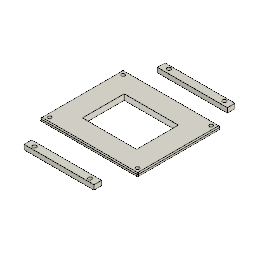
LCD Bezel 2.4in clamp-down v2 (Autodesk Fusion 360 design; units mm, degrees)
Autodesk Fusion 360 part; units mm, degrees
note: some values were not read from the file. Set by a fixed rule: which sketch regions a step uses.
sketch "Sketch1" plane through (0, 0, 0) normal (0, 0, 1) x (1, 0, 0)
  line L0 (-50.5, 43) -> (50.5, 43)
  line L1 (50.5, 43) -> (50.5, -43)
  line L2 (50.5, -43) -> (-50.5, -43)
  line L3 (-50.5, -43) -> (-50.5, 43)
  line L4 (-50.5, 43) -> (50.5, -43) construction
  line L5 (50.5, 43) -> (-50.5, -43) construction
  line L6 (25, 18.6) -> (-25, 18.6)
  line L7 (-25, 18.6) -> (-25, -18.6)
  line L8 (-25, -18.6) -> (25, -18.6)
  line L9 (25, -18.6) -> (25, 18.6)
  line L10 (25, 18.6) -> (-25, -18.6) construction
  line L11 (-25, 18.6) -> (25, -18.6) construction
  circle A0 centre (-45.5, 38) radius 5 construction
  circle A1 centre (-45.5, 38) radius 1.815
  line L12 (0, 55) -> (0, -45) construction
  line L13 (-60, 0) -> (80, 0) construction
  circle A2 centre (45.5, 38) radius 1.815
  circle A3 centre (45.5, -38) radius 1.815
  circle A4 centre (-45.5, -38) radius 1.815
  dimension "d1" = 101
  dimension "d2" = 86
  dimension "d3" = 50
  dimension "d4" = 37.2
  dimension "d5" = 5
  dimension "d6" = 3.63
  constraint perpendicular L0 L1
  constraint parallel L0 L2
  constraint parallel L1 L3
  constraint horizontal L0
  constraint coincident L4 origin
  constraint coincident L5 origin
  constraint perpendicular L6 L7
  constraint parallel L6 L8
  constraint parallel L7 L9
  constraint horizontal L6
  constraint coincident L10 origin
  constraint coincident L11 origin
  constraint tangent L3 A0
  constraint tangent L0 A0
  constraint concentric A0 A1
  constraint perpendicular L2 L12
  constraint perpendicular L3 L13
  constraint symmetric A1 L12 A2
  constraint symmetric A1 L13 A4
  constraint symmetric L13 A2 A3
  measures "d1" distance of L1.end L2.end
  measures "d2" distance of L0.end L1.end
  measures "d3" distance of L7.end L8.end
  measures "d4" distance of L6.end L7.end
  measures "d5" radius of A0
  measures "d6" diameter of A1
  measures "d14" distance of L0.start
extrude "Extrude1" add sketch "Sketch1" along normal blind 3 makes body 1
chamfer "Chamfer1" distance 3 angle 45 4 edges at (-25, 0, 3) (0, 18.6, 3) (25, 0, 3) (0, -18.6, 3) on bodies 1
sketch "Sketch2" plane through (-50.5, 0, 0) normal (-1, 0, 0) x (0, -1, 0)
  line L0 (-43, 0) -> (43, 0)
  line L1 (43, 0) -> (43, 3)
  line L2 (43, 3) -> (-43, 3)
  line L3 (-43, 3) -> (-43, 0)
fillet "Fillet1" radius 1 3 edges at (0, -43, 3) (0, 43, 3) (50.5, 0, 3) on bodies 1
sketch "Sketch3" plane through (0, 0, 0) normal (0, 0, 1) x (1, 0, 0)
  line L0 (-25.3857, -13.813) -> (-25.3857, 46.187) construction
  line L1 (25, 18.6) -> (25, -18.6)
  line L2 (25, -13.1739) -> (25, 45.4) construction
  line L3 (-34.2857, 33.1645) -> (-34.2857, -36.2651) construction
  line L4 (38.2, 40.4) -> (38.2, -34.6) construction
  line L5 (-25.3857, 18.7093) -> (64.6852, 18.7093) construction
  line L6 (60, 27.4093) -> (56.9479, 27.4093) construction
  line L7 (56.9479, 27.4093) -> (-67.0893, 27.4093) construction
  line L8 (60, -25.5) -> (-63.5008, -25.5) construction
  line L9 (25, -18.6) -> (-75, -18.6) construction
  line L10 (-34.2857, 0) -> (-38.2857, 0)
  line L11 (-38.2857, 0) -> (-38.2857, -5)
  line L12 (-38.2857, -5) -> (-34.2857, -5)
  line L13 (-34.2857, -5) -> (-34.2857, 0)
  line L14 (-34.2857, 0) -> (-38.2857, 0)
  line L15 (-38.2857, 0) -> (-38.2857, 5)
  line L16 (-38.2857, 5) -> (-34.2857, 5)
  line L17 (-34.2857, 5) -> (-34.2857, 0)
  line L18 (38.2, -25.5) -> (42.2, -25.5)
  line L19 (42.2, -25.5) -> (42.2, -10.5)
  line L20 (42.2, -10.5) -> (38.2, -10.5)
  line L21 (38.2, -10.5) -> (38.2, -25.5)
  line L22 (38.2, 27.4093) -> (42.2, 27.4093)
  line L23 (42.2, 27.4093) -> (42.2, 12.4093)
  line L24 (42.2, 12.4093) -> (38.2, 12.4093)
  line L25 (38.2, 12.4093) -> (38.2, 27.4093)
  line L26 (-34.2857, 27.4093) -> (-19.2857, 27.4093)
  line L27 (-19.2857, 27.4093) -> (-19.2857, 34.4093)
  line L28 (-19.2857, 34.4093) -> (-34.2857, 34.4093)
  line L29 (-34.2857, 34.4093) -> (-34.2857, 27.4093)
  line L30 (38.2, 27.4093) -> (23.2, 27.4093)
  line L31 (23.2, 27.4093) -> (23.2, 34.4093)
  line L32 (23.2, 34.4093) -> (38.2, 34.4093)
  line L33 (38.2, 34.4093) -> (38.2, 27.4093)
  line L34 (-34.2857, -25.5) -> (-19.2857, -25.5)
  line L35 (-19.2857, -25.5) -> (-19.2857, -32.5)
  line L36 (-19.2857, -32.5) -> (-34.2857, -32.5)
  line L37 (-34.2857, -32.5) -> (-34.2857, -25.5)
  line L38 (38.2, -25.5) -> (23.2, -25.5)
  line L39 (23.2, -25.5) -> (23.2, -32.5)
  line L40 (23.2, -32.5) -> (38.2, -32.5)
  line L41 (38.2, -32.5) -> (38.2, -25.5)
  line L42 (38.2, -25.5) -> (42.2, -25.5)
  line L43 (42.2, -25.5) -> (42.2, -30.5)
  line L44 (40.2, -32.5) -> (38.2, -32.5)
  line L45 (38.2, -32.5) -> (38.2, -25.5)
  line L46 (38.2, 27.4093) -> (42.2, 27.4093)
  line L47 (42.2, 27.4093) -> (42.2, 32.4093)
  line L48 (40.2, 34.4093) -> (38.2, 34.4093)
  line L49 (38.2, 34.4093) -> (38.2, 27.4093)
  line L50 (55, 0) -> (-65, 0) construction
  arc A0 (42.2, 32.4093) -> (40.2, 34.4093) centre (40.2, 32.4093) ccw
  arc A1 (40.2, -32.5) -> (42.2, -30.5) centre (40.2, -30.5) ccw
  dimension "d11" = 8.9
  dimension "d12" = 13.2
  dimension "d13" = 8.7
  dimension "d14" = 6.9
  dimension "d18" = 4
  dimension "d19" = 4
  dimension "d20" = 15
  dimension "d21" = 15
  dimension "d22" = 4
  dimension "d24" = 15
  dimension "d25" = 7
  dimension "d26" = 15
  dimension "d27" = 15
  dimension "d28" = 7
  dimension "d29" = 15
  dimension "d30" = 7
  dimension "d31" = 7
  dimension "d32" = 4
  dimension "d33" = 4
  dimension "d34" = 7
  dimension "d61" = 7
  dimension "d67" = 124.0372
  dimension "d75" = 2
  dimension "d76" = 2
  dimension "d79" = 4
  constraint vertical L0
  constraint coincident L1 L2.start
  constraint parallel L1 L2
  constraint vertical L3
  constraint vertical L4
  constraint coincident L0 L5.start
  constraint perpendicular L0 L5
  constraint horizontal L6
  constraint parallel L6 L7
  constraint horizontal L8
  constraint coincident L1.end L9.start
  constraint perpendicular L1 L9
  constraint horizontal L10
  constraint vertical L11
  constraint horizontal L12
  constraint vertical L13
  constraint coincident L3 L10.start
  constraint horizontal L14
  constraint vertical L15
  constraint horizontal L16
  constraint vertical L17
  constraint horizontal L18
  constraint vertical L19
  constraint horizontal L20
  constraint vertical L21
  constraint coincident L4 L18.start
  constraint coincident L8 L18.start
  constraint horizontal L22
  constraint vertical L23
  constraint horizontal L24
  constraint vertical L25
  constraint coincident L4 L22.start
  constraint coincident L7 L22.start
  constraint horizontal L26
  constraint vertical L27
  constraint horizontal L28
  constraint vertical L29
  constraint coincident L3 L26.start
  constraint coincident L7 L26.start
  constraint horizontal L30
  constraint vertical L31
  constraint horizontal L32
  constraint vertical L33
  constraint horizontal L34
  constraint vertical L35
  constraint horizontal L36
  constraint vertical L37
  constraint coincident L3 L34.start
  constraint coincident L8 L34.start
  constraint horizontal L38
  constraint vertical L39
  constraint horizontal L40
  constraint vertical L41
  constraint horizontal L42
  constraint vertical L43
  constraint horizontal L44
  constraint vertical L45
  constraint horizontal L46
  constraint vertical L47
  constraint horizontal L48
  constraint vertical L49
  constraint horizontal L50
  constraint tangent L47 A0
  constraint tangent L48 A0
  constraint tangent L44 A1
  constraint tangent L43 A1
  measures "d11" distance of L0 L3
  measures "d12" distance of L2 L4
  measures "d13" distance of L5 L7
  measures "d14" distance of L8 L9
  measures "d18" distance of L10.start L10.end
  measures "d19" distance of L18.start L18.end
  measures "d20" distance of L18.start L20.end
  measures "d21" distance of L22.start L24.end
  measures "d22" distance of L22.start L22.end
  measures "d24" distance of L26.start L26.end
  measures "d25" distance of L22.start L32.end
  measures "d26" distance of L22.start L30.end
  measures "d27" distance of L34.start L34.end
  measures "d28" distance of L34.start L36.end
  measures "d29" distance of L18.start L38.end
  measures "d30" distance of L18.start L40.end
  measures "d31" distance of L18.start L40.end
  measures "d32" distance of L18.start L18.end
  measures "d33" distance of L22.start L22.end
  measures "d34" distance of L22.start L32.end
  measures "d61" distance of L26 L28
  measures "d67" distance of L6.end L7.end
  measures "d75" radius of A0
  measures "d76" radius of A1
  measures "d79" distance of L3 L11
extrude "Extrude2" add sketch "Sketch3" against normal blind 6.2 bodies 1
fillet "Fillet2" radius 1 2 edges at (50.5, 43, 1) (50.2071, 42.7071, 2.7071) on bodies 1
fillet "Fillet3" radius 1 2 edges at (50.5, -43, 1) (50.2071, -42.7071, 2.7071) on bodies 1
sketch "Sketch4" plane through (0, -25.5, 0) normal (0, 1, 0) x (-1, 0, 0)
  line L0 (-23.2, 0) -> (-38.2, 0)
  line L1 (-38.2, 0) -> (-38.2, -6.2)
  line L2 (-38.2, -6.2) -> (-23.2, -6.2)
  line L3 (-23.2, -6.2) -> (-23.2, 0)
  line L4 (-23.2, -6.2) -> (-38.2, -6.2)
  line L5 (-38.2, -6.2) -> (-38.2, -3.2)
  line L6 (-38.2, -3.2) -> (-23.2, -3.2)
  line L7 (-23.2, -3.2) -> (-23.2, -6.2)
  dimension "d40" = 3
  constraint horizontal L4
  constraint vertical L5
  constraint horizontal L6
  constraint vertical L7
  constraint coincident L2.end L3.start
  measures "d40" distance of L2.end L6.end
fillet "Fillet4" radius 1 5 edges at (-50.5, 43, 1) (-50.5, 42.7071, 2.7071) (-50.5, 0, 3) (-50.5, -42.7071, 2.7071) (-50.5, -43, 1) on bodies 1
sketch "Sketch5" plane through (0, -25.5, 0) normal (0, 1, 0) x (-1, 0, 0)
  line L0 (34.2857, 0) -> (19.2857, 0)
  line L1 (19.2857, 0) -> (19.2857, -6.2)
  line L2 (19.2857, -6.2) -> (34.2857, -6.2)
  line L3 (34.2857, -6.2) -> (34.2857, 0)
  line L4 (34.2857, -6.2) -> (19.2857, -6.2)
  line L5 (19.2857, -6.2) -> (19.2857, -3.2)
  line L6 (19.2857, -3.2) -> (34.2857, -3.2)
  line L7 (34.2857, -3.2) -> (34.2857, -6.2)
  circle A0 centre (27.0136, -7.0821) radius 1090.7798
  dimension "d43" = 3
  constraint horizontal L4
  constraint vertical L5
  constraint horizontal L6
  constraint vertical L7
  constraint coincident L2.end L3.start
  measures "d43" distance of L2.end L6.end
sketch "Sketch6" plane through (0, 27.4093, 0) normal (0, -1, 0) x (1, 0, 0)
  line L0 (-19.2857, 0) -> (-34.2857, 0)
  line L1 (-34.2857, 0) -> (-34.2857, -6.2)
  line L2 (-34.2857, -6.2) -> (-19.2857, -6.2)
  line L3 (-19.2857, -6.2) -> (-19.2857, 0)
  line L4 (-19.2857, -6.2) -> (-34.2857, -6.2)
  line L5 (-34.2857, -6.2) -> (-34.2857, -3.2)
  line L6 (-34.2857, -3.2) -> (-19.2857, -3.2)
  line L7 (-19.2857, -3.2) -> (-19.2857, -6.2)
  dimension "d46" = 3
  constraint horizontal L4
  constraint vertical L5
  constraint horizontal L6
  constraint vertical L7
  constraint coincident L1 L5.end
  constraint coincident L2.end L3.start
  measures "d46" distance of L2.end L6.end
sketch "Sketch8" plane through (0, 0, -6.2) normal (0, 0, -1) x (1, 0, 0)
  line L0 (38.2, 25.5) -> (37.2, 25.5)
  line L1 (37.2, 25.5) -> (37.2, 29.5)
  line L2 (37.2, 29.5) -> (38.2, 29.5)
  line L3 (38.2, 29.5) -> (38.2, 25.5)
  line L4 (42.2, 10.5) -> (42.2, 30.5)
  arc A0 (42.2, 30.5) -> (40.2, 32.5) centre (40.2, 30.5) ccw
  line L5 (40.2, 32.5) -> (23.2, 32.5)
  line L6 (23.2, 32.5) -> (23.2, 25.5)
  line L7 (23.2, 25.5) -> (38.2, 25.5)
  line L8 (38.2, 25.5) -> (38.2, 10.5)
  line L9 (38.2, 10.5) -> (42.2, 10.5)
  dimension "d52" = 1
  constraint horizontal L0
  constraint vertical L1
  constraint horizontal L2
  constraint vertical L3
  measures "d52" distance of L0.start L0.end
sketch "Sketch10" plane through (0, 27.4093, 0) normal (0, -1, 0) x (1, 0, 0)
  line L0 (38.2, 0) -> (23.2, 0)
  line L1 (23.2, 0) -> (23.2, -6.2)
  line L2 (23.2, -6.2) -> (38.2, -6.2)
  line L3 (23.2, -6.2) -> (37.2, -6.2)
  line L4 (37.2, -6.2) -> (37.2, -3.2)
  line L5 (37.2, -3.2) -> (23.2, -3.2)
  line L6 (23.2, -3.2) -> (23.2, -6.2)
  line L7 (38.2, -6.2) -> (38.2, 0)
  dimension "d58" = 3
  constraint horizontal L3
  constraint vertical L4
  constraint horizontal L5
  constraint vertical L6
  constraint coincident L1.end L2.start
  measures "d58" distance of L1.end L5.end
sketch "Sketch11" plane through (0, 0, 0) normal (0, 0, -1) x (1, 0, 0)
  line L0 (42.2, 30.5) -> (42.2, 10.5)
  line L1 (42.2, 10.5) -> (38.2, 10.5)
  line L2 (38.2, 10.5) -> (38.2, 25.5)
  line L3 (38.2, -27.4093) -> (38.2, -12.4093)
  line L4 (38.2, -12.4093) -> (42.2, -12.4093)
  line L5 (42.2, -12.4093) -> (42.2, -32.4093)
  line L6 (40.2, -34.4093) -> (23.2, -34.4093)
  arc A0 (-50.5, -42) -> (-49.5, -43) centre (-49.5, -42) ccw
  line L7 (-49.5, -43) -> (49.5, -43)
  arc A1 (49.5, -43) -> (50.5, -42) centre (49.5, -42) ccw
  line L8 (50.5, -42) -> (50.5, 42)
  arc A2 (50.5, 42) -> (49.5, 43) centre (49.5, 42) ccw
  line L9 (49.5, 43) -> (-49.5, 43)
  arc A3 (-49.5, 43) -> (-50.5, 42) centre (-49.5, 42) ccw
  line L10 (-50.5, 42) -> (-50.5, -42)
  line L11 (-38.2857, 5) -> (-34.2857, 5)
  line L12 (-34.2857, 5) -> (-34.2857, -5)
  line L13 (-34.2857, -5) -> (-38.2857, -5)
  line L14 (-38.2857, -5) -> (-38.2857, 5)
  line L15 (-19.2857, 32.5) -> (-19.2857, 25.5)
  line L16 (-19.2857, 25.5) -> (-34.2857, 25.5)
  line L17 (-34.2857, 25.5) -> (-34.2857, 32.5)
  line L18 (-34.2857, 32.5) -> (-19.2857, 32.5)
  line L19 (-34.2857, -27.4093) -> (-19.2857, -27.4093)
  line L20 (-19.2857, -27.4093) -> (-19.2857, -34.4093)
  line L21 (-19.2857, -34.4093) -> (-34.2857, -34.4093)
  line L22 (-34.2857, -34.4093) -> (-34.2857, -27.4093)
  line L23 (38.2, 25.5) -> (23.2, 25.5)
  line L24 (23.2, 25.5) -> (23.2, 32.5)
  line L25 (23.2, 32.5) -> (40.2, 32.5)
  line L26 (23.2, -34.4093) -> (23.2, -27.4093)
  line L27 (23.2, -27.4093) -> (38.2, -27.4093)
  circle A4 centre (-45.5, 38) radius 1.815
  line L28 (25, 18.6) -> (25, -18.6)
  line L29 (25, -18.6) -> (-25, -18.6)
  line L30 (-25, -18.6) -> (-25, 18.6)
  line L31 (-25, 18.6) -> (25, 18.6)
  circle A5 centre (45.5, 38) radius 1.815
  circle A6 centre (-45.5, -38) radius 1.815
  circle A7 centre (45.5, -38) radius 1.815
  line L32 (38.2, 10.5) -> (38.2, -12.4093) construction
  arc A8 (42.2, 30.5) -> (40.2, 32.5) centre (40.2, 30.5) ccw
  arc A9 (40.2, -34.4093) -> (42.2, -32.4093) centre (40.2, -32.4093) ccw
  constraint coincident L1.end L2.start
  constraint coincident L3.end L4.start
sketch "Sketch12" plane through (0, 0, -6.2) normal (0, 0, -1) x (1, 0, 0)
  line L0 (-19.2857, 25.5) -> (-19.2857, 32.5)
  line L1 (-19.2857, 32.5) -> (-34.2857, 32.5)
  line L2 (-34.2857, 32.5) -> (-34.2857, 25.5)
  circle A0 centre (-26.7857, 29) radius 1.75
  line L3 (0, -45) -> (0, 45) construction
  line L4 (-19.2857, 25.5) -> (-19.2857, 32.5)
  circle A1 centre (30.7, 29) radius 1.75
  line L5 (23.2, 32.5) -> (38.2, 32.5)
  line L6 (-19.2857, 32.5) -> (-34.2857, 32.5)
  circle A2 centre (-26.7857, -30.9093) radius 1.75
  circle A3 centre (30.7, -30.9093) radius 1.75
  line L7 (-34.2857, -27.4093) -> (-19.2857, -27.4093)
  line L8 (23.2, -27.4093) -> (37.2, -27.4093)
  line L9 (-19.2857, -27.4093) -> (-19.2857, -34.4093)
  line L10 (23.2, -27.4093) -> (23.2, -34.4093)
  line L11 (-34.2857, 25.5) -> (-19.2857, 25.5)
  line L12 (-26.7857, -30.9093) -> (-26.7857, 47.6742) construction
  line L13 (30.7, -30.9093) -> (30.7, 41.2834) construction
  line L14 (23.2, 25.5) -> (23.2, 32.5) construction
  dimension "d80" = 3.5
  dimension "d81" = 7.5
  dimension "d82" = 3.5
  dimension "d83" = 3.5
  dimension "d84" = 3.5
  dimension "d85" = 3.5
  dimension "d86" = 3.5
  dimension "d87" = 3.5
  dimension "d88" = 3.5
  dimension "d89" = 7.5
  dimension "d90" = 7.5
  dimension "d109" = 7.5
  constraint vertical L3
  constraint coincident A2.centre L12.start
  constraint perpendicular L7 L12
  constraint coincident A3.centre L13.start
  constraint perpendicular L5 L13
  measures "d80" diameter of A0
  measures "d81" distance of A0.centre L4
  measures "d82" diameter of A1
  measures "d83" distance of A1.centre L5
  measures "d84" distance of A0.centre L6
  measures "d85" diameter of A2
  measures "d86" diameter of A3
  measures "d87" distance of A2.centre L7
  measures "d88" distance of A3.centre L8
  measures "d89" distance of A2.centre L9
  measures "d90" distance of A3.centre L10
  measures "d109" distance of A1.centre L14
sketch "Sketch1 (2)" plane through (0, 0, 0) normal (0, 0, 1) x (1, 0, 0) in component "Clamp"
  line L0 (-34.1545, -32.6158) -> (37.4777, -32.6158)
  line L1 (37.4777, -32.6158) -> (37.4777, -24.6158)
  line L2 (37.4777, -24.6158) -> (-34.1545, -24.6158)
  line L3 (-34.1545, -24.6158) -> (-34.1545, -32.6158)
  dimension "d110" = 8
  constraint horizontal L0
  constraint vertical L1
  constraint horizontal L2
  constraint vertical L3
  measures "d110" distance of L0.start L2.end
copy_body "Body->Comp1" bodies 1 removing the originals makes body 2 in component "Bezel"
sketch "Sketch1 (3)" plane through (0, 0, -6.2) normal (0, 0, -1) x (1, 0, 0) in component "Bezel"
  line L0 (38.2, -12.4093) -> (38.2, -27.4093)
  line L1 (38.2, -27.4093) -> (23.2, -27.4093)
  line L2 (23.2, -27.4093) -> (23.2, -34.4093)
  line L3 (23.2, -34.4093) -> (40.2, -34.4093)
  arc A0 (40.2, -34.4093) -> (42.2, -32.4093) centre (40.2, -32.4093) ccw
  line L4 (42.2, -32.4093) -> (42.2, -12.4093)
  line L5 (42.2, -12.4093) -> (38.2, -12.4093)
  circle A1 centre (-26.7857, 29) radius 1.75
  line L6 (-19.2857, 32.5) -> (-34.2857, 32.5)
  circle A2 centre (30.7, 29) radius 1.75
  line L7 (23.2, 32.5) -> (38.2, 32.5)
  line L8 (-34.2857, -33.1645) -> (-34.2857, 36.2651)
  line L9 (38.2, 32.5) -> (38.2, 25.5)
  line L10 (-26.7857, 29) -> (-26.7857, -48.7711) construction
  line L11 (30.7, 29) -> (30.7, -48.399) construction
  circle A3 centre (-26.7857, -30.9093) radius 1.75
  line L12 (-19.2857, -34.4093) -> (-34.2857, -34.4093)
  circle A4 centre (30.7, -30.9093) radius 1.75
  line L13 (23.2, -34.4093) -> (38.2, -34.4093)
  line L14 (-34.692, -70.5362) -> (37.808, -70.5362)
  line L15 (37.808, -70.5362) -> (37.808, -62.5362)
  line L16 (37.808, -62.5362) -> (-34.692, -62.5362)
  line L17 (-34.692, -62.5362) -> (-34.692, -70.5362)
  line L18 (-41.389, -67.0362) -> (51.2524, -67.0362) construction
  circle A5 centre (-27.192, -67.0362) radius 2
  circle A6 centre (30.308, -67.0362) radius 2
  dimension "d111" = 3.5
  dimension "d112" = 3.5
  dimension "d113" = 3.5
  dimension "d114" = 3.5
  dimension "d115" = 7.5
  dimension "d116" = 7.5
  dimension "d117" = 57.4857
  dimension "d118" = 3.5
  dimension "d119" = 3.5
  dimension "d120" = 3.5
  dimension "d121" = 3.5
  dimension "d124" = 72.5
  dimension "d125" = 8
  dimension "d126" = 3.5
  dimension "d127" = 4
  dimension "d128" = 7.5
  dimension "d129" = 4
  dimension "d130" = 57.5
  constraint coincident A1.centre L10.start
  constraint vertical L10
  constraint coincident A2.centre L11.start
  constraint perpendicular L1 L11
  constraint coincident L10 A3.centre
  constraint coincident L11 A4.centre
  constraint horizontal L14
  constraint vertical L15
  constraint horizontal L16
  constraint vertical L17
  constraint perpendicular L15 L18
  constraint coincident L18 A5.centre
  constraint coincident L18 A6.centre
  measures "d111" diameter of A1
  measures "d112" distance of A1.centre L6
  measures "d113" diameter of A2
  measures "d114" distance of A2.centre L7
  measures "d115" distance of A1.centre L8
  measures "d116" distance of A2.centre L9
  measures "d117" distance of A1.centre A2.centre
  measures "d118" diameter of A3
  measures "d119" distance of A3.centre L12
  measures "d120" diameter of A4
  measures "d121" distance of A4.centre L13
  measures "d124" distance of L14.start L14.end
  measures "d125" distance of L14.start L16.end
  measures "d126" distance of L14 L18
  measures "d127" diameter of A5
  measures "d128" distance of L17 A5.centre
  measures "d129" diameter of A6
  measures "d130" distance of A5.centre A6.centre
extrude "Extrude2'" add sketch "Sketch1 (3)" along normal blind 5 separate body contours L14 L15 L16 L17 makes body 3 in component "Bezel"
extrude "Extrude1'" cut sketch "Sketch1 (3)" against normal blind 6 contours A1 | A2 | A3 | A4 bodies 2 in component "Bezel"
move_body "Move1" bodies 3 to x (-1, 0, 0) y (0, -1, 0) z (0, 0, 1) at (-69.384, -4.9276, 0) in component "Bezel"
move_body "Move2" bodies 3 to x (1, 0, 0) y (0, 1, 0) z (0, 0, 1) at (72.5, 0, 0) in component "Bezel"
extrude "Extrude13" add sketch "Sketch1 (3)" along normal blind 5 separate body contours L14 L15 L16 L17 makes body 4
move_body "Align1" bodies 4 to x (1, 0, 0) y (0, 1, 0) z (0, 0, 1) at (0, 0, 6.2)
move_body "Align1'" bodies 3 to x (1, 0, 0) y (0, 1, 0) z (0, 0, 1) at (0, 0, 6.2) in component "Bezel"
move_body "Align2" bodies 2 to x (1, 0, 0) y (0, 1, 0) z (0, 0, 1) at (0, 0, -3) in component "Bezel"
extrude "Extrude11" [suppressed]
sketch "Sketch7" plane through (0, 0, -6.2) normal (0, 0, -1) x (1, 0, 0)
  line L0 (38.2, -27.4093) -> (37.2, -27.4093)
  line L1 (37.2, -27.4093) -> (37.2, -31.4093)
  line L2 (37.2, -31.4093) -> (38.2, -31.4093)
  line L3 (38.2, -31.4093) -> (38.2, -27.4093)
  circle A0 centre (30.7, -30.9093) radius 1.75
  line L4 (38.2, -12.4093) -> (38.2, -27.4093)
  line L5 (38.2, -27.4093) -> (23.2, -27.4093)
  line L6 (23.2, -27.4093) -> (23.2, -34.4093)
  line L7 (23.2, -34.4093) -> (40.2, -34.4093)
  arc A1 (40.2, -34.4093) -> (42.2, -32.4093) centre (40.2, -32.4093) ccw
  line L8 (42.2, -32.4093) -> (42.2, -12.4093)
  line L9 (42.2, -12.4093) -> (38.2, -12.4093)
  dimension "d49" = 1
  constraint horizontal L0
  constraint vertical L1
  constraint horizontal L2
  constraint vertical L3
  measures "d49" distance of L0.start L0.end
component "Clamp" placed x (1, 0, 0) y (0, 1, 0) z (0, 0, 1) at (0, 0, 0)
component "Bezel" placed x (1, 0, 0) y (0, 1, 0) z (0, 0, 1) at (0, 0, 0)
named bodies: "Bezel", "clip", "Duplicate clip"
